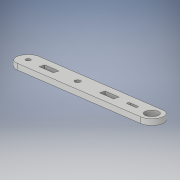
# Autodesk Inventor part: 連接3
Saved by Autodesk Inventor 2017 (Build 210142000, 142)
## iProperties
Part Number: 連接3
Material: 一般
Document SubType Name: Modeling
Designer: User
Density: 1 g/cm^3
Appearance: 預設
Author: User
Autodesk Inventor part; units mm, degrees
ref_plane "YZ Plane" through (0, 0, 0) normal (1, 0, 0) x (0, 1, 0)
ref_plane "XZ Plane" through (0, 0, 0) normal (0, 1, 0) x (-1, 0, 0)
ref_plane "XY Plane" through (0, 0, 0) normal (0, 0, 1) x (1, 0, 0)
sketch "草圖1" plane through (0, 0, 0) normal (0, 1, 0) x (-1, 0, 0)
  circle A0 centre (0, 0) radius 1.25
  line L0 (0, 0) -> (-80, 0)
  circle A1 centre (-80, 0) radius 3.6
  circle A2 centre (-80, 0) radius 6
  circle A3 centre (0, 0) radius 6
  line L1 (0, 6) -> (-80, 6)
  line L2 (-80, -6) -> (0, -6)
  dimension "d0" = 2.5
  dimension "d14" = 80
  dimension "d15" = 7.2
  dimension "d16" = 12
  dimension "d17" = 12
  constraints: 6 end point, 4 centre point, 4 coincident, 4 point on circle, 2 horizontal, 1 tangent
  measures "d0" diameter of A0
  measures "d14" distance of L0.start L0.end
  measures "d15" diameter of A1
  measures "d16" diameter of A2
  measures "d17" diameter of A3
extrude "擠出1" add sketch "草圖1" along normal mid plane 3
sketch "草圖2" plane through (0, 1.5, 0) normal (0, 1, 0) x (1, 0, 0)
  circle A0 centre (80, 0) radius 3.6 projected
  circle A1 centre (0, 0) radius 1.25 projected
  arc A2 (0, 6) -> (0, -6) centre (0, 0) ccw projected
  line L0 (0, -6) -> (80, -6) projected
  arc A3 (80, -6) -> (80, 6) centre (80, 0) ccw projected
  line L1 (80, 6) -> (0, 6) projected
  line L2 (80, 0) -> (70, 0)
  line L3 (70, 0) -> (65, 0) construction
  line L4 (70, 0.75) -> (65, 0.75)
  line L5 (65, -0.75) -> (70, -0.75)
  arc A4 (70, -0.75) -> (70, 0.75) centre (70, 0) ccw
  arc A5 (65, 0.75) -> (65, -0.75) centre (65, 0) ccw
  line L6 (65, 0) -> (57, 0)
  line L7 (57, 0) -> (57, 1.5)
  line L8 (57, 1.5) -> (48, 1.5)
  line L9 (48, 1.5) -> (48, -1.5)
  line L10 (48, -1.5) -> (57, -1.5)
  line L11 (57, -1.5) -> (57, 0)
  line L12 (48, 0) -> (32, 0)
  circle A6 centre (32, 0) radius 1.5
  line L13 (32, 0) -> (18, 0)
  line L14 (18, 0) -> (18, 1.5)
  line L15 (18, 1.5) -> (9, 1.5)
  line L16 (9, 1.5) -> (9, -1.5)
  line L17 (9, -1.5) -> (18, -1.5)
  line L18 (18, -1.5) -> (18, 0)
  point P0 (67.5, 0)
  dimension "d18" = 10
  dimension "d19" = 5
  dimension "d20" = 1.5
  dimension "d21" = 8
  dimension "d22" = 1.5
  dimension "d23" = 9
  dimension "d24" = 3
  dimension "d25" = 16
  dimension "d27" = 3
  dimension "d28" = 14
  dimension "d29" = 1.5
  dimension "d30" = 9
  dimension "d31" = 3
  constraints: 36 end point, 9 perpendicular, 5 horizontal, 4 point on circle, 4 tangent, 3 centre point, 2 midpoint, 2 point on line, 1 coincident, 1 parallel
  measures "d18" distance of L2.start L2.end
  measures "d19" distance of L2.end L3.end
  measures "d20" diameter of A5
  measures "d21" distance of L3.end L6.end
  measures "d22" distance of L6.end L7.end
  measures "d23" distance of L7.end L8.end
  measures "d24" distance of L8.end L9.end
  measures "d25" distance of L12.start L12.end
  measures "d27" diameter of A6
  measures "d28" distance of L13.start L13.end
  measures "d29" distance of L18.end L15.start
  measures "d30" distance of L15.start L16.start
  measures "d31" distance of L16.start L16.end
extrude "擠出2" cut sketch "草圖2" against normal blind 10 contours L18 L17 L16 L15 L14 | A6 L13 L12 | L12 L13 A6 | L11 L10 L9 L8 L7 | A4 L5 A5 L4
